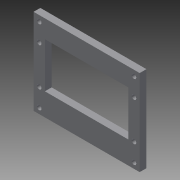
# Autodesk Inventor part: ProxSensor_Bracket_Back
Saved by Autodesk Inventor 2015 (Build 190159000, 159)
## iProperties
Created: 2015-03-05
Part Number: ProxSensor_Bracket_Back
Material: Generic
Document SubType Name: Modeling
Designer: ChristopherEvan
Density: 1 g/cm^3
Appearance: Default
Author: ChristopherEvan
Autodesk Inventor part; units mm, degrees
ref_plane "YZ Plane" through (0, 0, 0) normal (1, 0, 0) x (0, 1, 0)
ref_plane "XZ Plane" through (0, 0, 0) normal (0, 1, 0) x (-1, 0, 0)
ref_plane "Work Plane1" through (0, 0, 0) normal (0, 0, 1) x (1, 0, 0)
sketch "Sketch1" plane through (0, 0, 0) normal (0, 0, 1) x (1, 0, 0)
  circle A0 centre (2.5, -19.5) radius 1 projected
  circle A1 centre (2.5, -2.5) radius 1 projected
  circle A2 centre (44.5, -2.5) radius 1 projected
  circle A3 centre (44.5, -19.5) radius 1 projected
  line L0 (0, -25) -> (0, 3) projected
  line L1 (0, -25) -> (47, -25) projected
  line L2 (47, -25) -> (47, 3) projected
  line L3 (0, 3) -> (47, 3) projected
  line L4 (5, 0) -> (42, 0) projected
  line L5 (42, 0) -> (42, -20) projected
  line L6 (42, -20) -> (5, -20) projected
  line L7 (5, -20) -> (5, 0) projected
  point P0 (0, 0)
extrude "Extrusion1" add sketch "Sketch1" along normal blind 3
sketch "Sketch2" plane through (0, 0, 3) normal (0, 0, 1) x (1, 0, 0)
  line L0 (47, 3) -> (0, 3) projected
  line L1 (47, 3) -> (0, 3)
  line L2 (0, 3) -> (0, 8)
  line L3 (0, 8) -> (47, 8)
  line L4 (47, 8) -> (47, 3)
  line L5 (0, -25) -> (47, -25) projected
  line L6 (0, -25) -> (47, -25)
  line L7 (47, -25) -> (47, -30)
  line L8 (47, -30) -> (0, -30)
  line L9 (0, -30) -> (0, -25)
  point P0 (0, 0)
  dimension "d2" = 5
  dimension "d3" = 5
  constraints: 16 end point, 4 parallel, 2 horizontal, 2 perpendicular
  measures "d2" distance between parallel lines of L3 L1
  measures "d3" distance between parallel lines of L8 L5
extrude "Extrusion2" add sketch "Sketch2" against normal blind 3
sketch "Sketch4" plane through (0, 0, 3) normal (0, 0, 1) x (1, 0, 0)
  circle A0 centre (2.5, -2.5) radius 1 projected
  circle A1 centre (44.5, -2.5) radius 1 projected
  circle A2 centre (44.5, -19.5) radius 1 projected
  circle A3 centre (2.5, -19.5) radius 1 projected
  circle A4 centre (2.5, 5.5) radius 1
  circle A5 centre (44.5, 5.5) radius 1
  circle A6 centre (2.5, -27.5) radius 1
  circle A7 centre (44.5, -27.5) radius 1
  line L0 (0, 8) -> (47, 8) projected
  line L1 (47, -30) -> (0, -30) projected
  point P0 (0, 0)
  dimension "d6" = 2.5
  dimension "d7" = 2.5
  dimension "d8" = 2.5
  dimension "d9" = 2.5
  constraints: 4 centre point
  measures "d6" distance from line of L0 A5.centre
  measures "d7" distance from line of L0 A4.centre
  measures "d8" distance from line of L1 A6.centre
  measures "d9" distance from line of A7.centre L1
extrude "Extrusion3" cut sketch "Sketch4" against normal blind 3 contours A4 | A5 | A6 | A7
body "Solid1"
